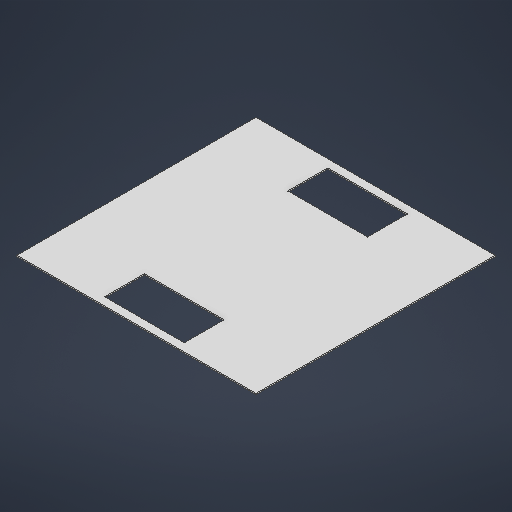
# Autodesk Inventor part: base 30x30
Saved by Autodesk Inventor 2027 (Build 310192060, 192F)
## iProperties
Created: 2026-09-04
Part Number: base 30x30
Material: Genérico
Document SubType Name: Modeling
Designer: Leandro
Density: 1 g/cm^3
Appearance: Valor por defecto
Author: Leandro
Autodesk Inventor part; units mm, degrees
ref_plane "YZ Plane" through (0, 0, 0) normal (1, 0, 0) x (0, 1, 0)
ref_plane "XZ Plane" through (0, 0, 0) normal (0, 1, 0) x (-1, 0, 0)
ref_plane "XY Plane" through (0, 0, 0) normal (0, 0, 1) x (1, 0, 0)
sketch "Boceto1" plane through (0, 0, 0) normal (0, 1, 0) x (-1, 0, 0)
  line L0 (16.7386, 18.54) -> (16.7386, -281.46)
  line L1 (16.7386, -281.46) -> (316.7386, -281.46)
  line L2 (316.7386, -281.46) -> (316.7386, 18.54)
  line L3 (316.7386, 18.54) -> (16.7386, 18.54)
  point P0 (0, 0)
  dimension "d2" = 300
  dimension "d3" = 300
  constraints: 8 end point, 3 perpendicular, 1 vertical
  measures "d2" distance of L0.start L0.end
  measures "d3" distance of L0.end L1.end
extrude "Extrusión1" add sketch "Boceto1" along normal mid plane 1.5
sketch "Boceto2" plane through (0, 0.75, 0) normal (0, 1, 0) x (1, 0, 0)
  line L0 (-316.7386, -18.54) -> (-16.7386, -18.54) projected
  line L1 (-16.7386, 281.46) -> (-316.7386, 281.46) projected
  line L2 (-316.7386, 281.46) -> (-316.7386, -18.54) projected
  line L3 (-316.7386, 131.46) -> (-16.7386, 131.46)
  line L4 (-16.7386, -18.54) -> (-16.7386, 281.46) projected
  line L5 (-166.7386, -18.54) -> (-166.7386, -8.54)
  line L6 (-166.7386, 281.46) -> (-166.7386, 271.46)
  line L7 (-166.7386, 271.46) -> (-116.7386, 271.46)
  line L8 (-116.7386, 271.46) -> (-116.7386, 221.46)
  line L9 (-116.7386, 221.46) -> (-166.7386, 221.46)
  line L10 (-166.7386, 221.46) -> (-216.7386, 221.46)
  line L11 (-216.7386, 221.46) -> (-216.7386, 271.46)
  line L12 (-216.7386, 271.46) -> (-166.7386, 271.46)
  line L13 (-166.7386, -8.54) -> (-216.7386, -8.54)
  line L14 (-216.7386, -8.54) -> (-216.7386, 41.46)
  line L15 (-216.7386, 41.46) -> (-166.7386, 41.46)
  line L16 (-116.7386, 41.46) -> (-166.7386, 41.46)
  line L17 (-116.7386, -8.54) -> (-166.7386, -8.54)
  line L18 (-116.7386, 41.46) -> (-116.7386, -8.54)
  line L19 (-166.7386, -18.54) -> (-166.7386, -8.54)
  line L20 (-166.7386, 271.46) -> (-166.7386, 281.46)
  point P0 (0, 0)
  dimension "d6" = 10
  dimension "d7" = 10
  dimension "d8" = 50
  dimension "d9" = 50
  dimension "d10" = 50
  dimension "d11" = 50
  dimension "d12" = 50
  constraints: 34 end point, 8 perpendicular, 4 midpoint, 3 horizontal, 2 point on line, 1 collinear, 1 vertical
  measures "d6" distance of L5.start L5.end
  measures "d7" distance of L6.end L6.start
  measures "d8" distance of L6.end L7.end
  measures "d9" distance of L7.end L8.end
  measures "d10" distance of L9.end L10.end
  measures "d11" distance of L5.end L13.end
  measures "d12" distance of L13.end L14.end
extrude "Extrusión2" cut sketch "Boceto2" against normal blind 4 contours L13 L14 L15 L16 L18 L17 | L7 L8 L9 L10 L11 L12
